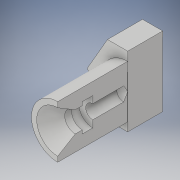
# Autodesk Inventor part: 示範一
Saved by Autodesk Inventor 2017 (Build 210142000, 142)
## iProperties
Part Number: 示範一
Material: 一般
Document SubType Name: Modeling
Designer: user
Density: 1 g/cm^3
Appearance: 預設
Author: user
Autodesk Inventor part; units mm, degrees
ref_plane "YZ Plane" through (0, 0, 0) normal (1, 0, 0) x (0, 1, 0)
ref_plane "XZ Plane" through (0, 0, 0) normal (0, 1, 0) x (-1, 0, 0)
ref_plane "XY Plane" through (0, 0, 0) normal (0, 0, 1) x (1, 0, 0)
sketch "草圖1" plane through (0, 0, 0) normal (1, 0, 0) x (0, 1, 0)
  line L0 (2, 1.1547) -> (2, 10)
  line L1 (2, 10) -> (4, 10)
  line L2 (4, 10) -> (4, 13)
  line L3 (3, 15) -> (6, 20)
  line L4 (6, 20) -> (7.5, 20)
  arc A0 (7.3358, 14.0988) -> (7.3358, 14.0988) centre (-51.8892, 10.8387) ccw
  line L5 (7.5, 20) -> (7.5, 0)
  line L6 (0, -10) -> (0, 12.2342)
  line L7 (4, 13) -> (3, 13)
  line L8 (3, 13) -> (3, 15)
  line L9 (2, 1.1547) -> (0, 0)
  line L10 (0, 0) -> (7.5, 0)
  dimension "d3" = 8
  dimension "d4" = 4
  dimension "d5" = 15
  dimension "d6" = 12
  dimension "d7" = 6
  dimension "d8" = 5
  dimension "d9" = 7
  dimension "d10" = 3
  dimension "d11" = 0
  dimension "d19" = 20
  dimension "d24" = 20
  dimension "d25" = 0
  dimension "d27" = 60
  constraints: 22 end point, 3 perpendicular, 3 vertical, 2 point on circle, 1 centre point, 1 horizontal, 1 point on line
  measures "d3" diameter of L2 L6
  measures "d4" diameter of L0 L6
  measures "d5" diameter of L5 L6
  measures "d6" diameter of L3.end L6
  measures "d7" diameter of L8 L6
  measures "d8" vertical distance of L3.start L3.end
  measures "d9" distance between parallel lines of L7 L4
  measures "d10" distance of L1.end L2.end
  measures "d11" distance from line of point (0, 0) L6
  measures "d19" distance from line of L9.end L4
  measures "d24" distance from line of L5.end L4
  measures "d25" distance from line of point (0, 0) L10
  measures "d27" angle of L9 L6
revolve "迴轉1" add sketch "草圖1" angle 180 about axis through (0, 0, -10) along (0, 0, 1) picked at (3.6603, 4.915) contours L0 L1 L2 L7 L8 L3 L4 A0 L10 L9 | A0 L4 L5 L10
sketch "草圖3" plane through (0, 0, 0) normal (0, 0, -1) x (-1, 0, 0)
  line L0 (0, -7.5) -> (0, 0) projected
  arc A0 (0, -7.5) -> (0, 7.5) centre (0, 0) ccw projected
  line L1 (-11.5773, 0) -> (12.4556, 0) construction
  line L2 (0.0279, 7.6444) -> (0.0279, -10.5735) construction
  line L3 (5.7735, 10) -> (11.547, 0)
  line L4 (11.547, 0) -> (5.7735, -10)
  line L5 (5.7735, -10) -> (0.0248, -10)
  line L6 (0, 10) -> (5.7735, 10)
  line L7 (-0.0017, 11.3448) -> (0.0279, -12.4793) construction
  line L8 (0.0248, -10) -> (0, 10)
  point P0 (6.4952, 3.75)
  dimension "d29" = 20
  dimension "d32" = 2.5
  constraints: 16 end point, 3 point on line, 2 coincident, 1 collinear, 1 horizontal, 1 point on circle, 1 vertical, 6 other
  measures "d29" distance between parallel lines of L6 L5
  measures "d32" distance from line of L6 A0.end
extrude "擠出1" add sketch "草圖3" along normal blind 10
